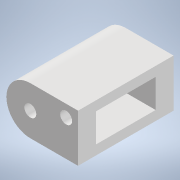
# Autodesk Inventor part: 3rd arm
Saved by Autodesk Inventor 2022 (Build 260153000, 153)
## iProperties
Created: 2021-06-30
Part Number: 3rd arm
Material: Generic
Document SubType Name: Modeling
Designer: USER
Density: 1 g/cm^3
Appearance: Default
Author: USER
Autodesk Inventor part; units mm, degrees
ref_plane "YZ Plane" through (0, 0, 0) normal (1, 0, 0) x (0, 1, 0)
ref_plane "XZ Plane" through (0, 0, 0) normal (0, 1, 0) x (-1, 0, 0)
ref_plane "XY Plane" through (0, 0, 0) normal (0, 0, 1) x (1, 0, 0)
sketch "Sketch1" plane through (0, 0, 0) normal (0, 0, 1) x (1, 0, 0)
  line L0 (-25, 10) -> (25, 10)
  line L1 (25, 10) -> (25, -10)
  line L2 (25, -10) -> (-25, -10)
  line L3 (-25, -10) -> (-25, 10)
  line L4 (-25, 10) -> (25, -10) construction
  line L5 (25, 10) -> (-25, -10) construction
  point P0 (0, 0)
  dimension "d0" = 50
  dimension "d1" = 20
  constraints: 12 end point, 2 midpoint, 2 parallel, 1 horizontal, 1 perpendicular
  measures "d0" distance of L1.end L2.end
  measures "d1" distance of L0.end L1.end
extrude "Extrusion1" add sketch "Sketch1" along normal blind 40
sketch "Sketch2" plane through (0, 0, 40) normal (0, 0, 1) x (1, 0, 0)
  circle A0 centre (-15, 0) radius 2.5
  line L0 (-25, 10) -> (-25, -10) projected
  line L1 (-25, -10) -> (25, -10) projected
  point P0 (0, 0)
  dimension "d4" = 5
  dimension "d5" = 10
  dimension "d6" = 10
  constraints: 1 centre point
  measures "d4" diameter of A0
  measures "d5" distance from line of L0 A0.centre
  measures "d6" distance from line of L1 A0.centre
extrude "Extrusion2" cut sketch "Sketch2" against normal through all
sketch "Sketch3" plane through (25, -10, 0) normal (1, 0, 0) x (0, 0, -1)
  line L0 (-32.5, 4) -> (-7.5, 4)
  line L1 (-7.5, 4) -> (-7.5, 16)
  line L2 (-7.5, 16) -> (-32.5, 16)
  line L3 (-32.5, 16) -> (-32.5, 4)
  line L4 (-32.5, 4) -> (-7.5, 16) construction
  line L5 (-7.5, 4) -> (-32.5, 16) construction
  point P0 (0, 10)
  point P1 (-20, 10)
  dimension "d9" = 25
  dimension "d10" = 12
  constraints: 12 end point, 2 midpoint, 2 parallel, 1 horizontal, 1 perpendicular
  measures "d9" distance of L2.end L1.end
  measures "d10" distance of L1.end L0.end
extrude "Extrusion3" cut sketch "Sketch3" against normal blind 44
full round fillet "Full Round Fillet1" first side at (10.3333, 6, 15.8333) centre faces at (-19, -2, 15.8333) second side at (10.3333, -6, 24.1667)
full round fillet "Full Round Fillet2" first side at (8.3333, 10, 13.3333) centre faces at (-25, 3.3333, 13.3333) second side at (-8.3333, -10, 13.3333)
sketch "Sketch4" plane through (25, -10, 0) normal (1, 0, 0) x (0, 0, -1)
  line L0 (-40, 0) -> (-40, 20) projected
  line L1 (0, 20) -> (0, 0) projected
  line L2 (-40, 20) -> (0, 20)
  line L3 (0, 20) -> (0, 0)
  line L4 (0, 0) -> (-40, 0)
  line L5 (-40, 0) -> (-40, 20)
  point P0 (0, 10)
  constraints: 8 end point, 2 parallel, 1 horizontal, 1 perpendicular
extrude "Extrusion4" cut sketch "Sketch4" against normal blind 20
sketch "Sketch5" plane through (0, 0, 40) normal (0, 0, 1) x (1, 0, 0)
  line L0 (5, 10) -> (-15, 10) projected
  line L1 (5, -10) -> (5, 10) projected
  point P0 (0, 0)
  point P1 (0, 5)
  dimension "d15" = 5
  dimension "d16" = 5
  measures "d15" distance from line of L0 point (0, 5)
  measures "d16" distance from line of L1 point (0, 5)
hole "Hole1" at (0, 5, 40) direction (0, 0, -1) diameter 5 end through all
body "Solid1"
